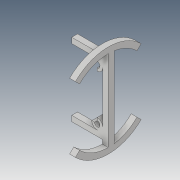
# Autodesk Inventor part: cameraMount2
Saved by Autodesk Inventor 2018 (Build 220112000, 112)
## iProperties
Created: 2020-02-12
Part Number: cameraMount2
Material: Generic
Document SubType Name: Modeling
Designer: anirudh.bali
Density: 1 g/cm^3
Appearance: Default
Author: anirudh.bali
Autodesk Inventor part; units mm, degrees
ref_plane "YZ Plane" through (0, 0, 0) normal (1, 0, 0) x (0, 1, 0)
ref_plane "XZ Plane" through (0, 0, 0) normal (0, 1, 0) x (-1, 0, 0)
ref_plane "XY Plane" through (0, 0, 0) normal (0, 0, 1) x (1, 0, 0)
sketch "Sketch2" plane through (0, 0, 0) normal (0, 0, 1) x (1, 0, 0)
  line L0 (0, 0) -> (40, 0)
  line L1 (40, 0) -> (40, 40)
  line L2 (40, 40) -> (0, 40)
  line L3 (0, 40) -> (0, 0)
  line L4 (0, 40) -> (2.5, 40)
  line L5 (40, 0) -> (37.5, 0)
  arc A0 (7.5046, 33.9954) -> (6.0046, 32.4954) centre (6.0046, 33.9954) ccw
  line L6 (6.0046, 32.4954) -> (6.0046, 30.9908)
  line L7 (7.5046, 33.9954) -> (9.0092, 33.9954)
  line L8 (0, 40) -> (3, 40)
  line L9 (40, 40) -> (37, 40)
  line L10 (0, 40) -> (3, 40)
  line L11 (40, 0) -> (37, 0)
  line L12 (6.0046, 37) -> (33.9954, 37)
  line L13 (37, 33.9954) -> (37, 6.0046)
  line L14 (33.9954, 3) -> (6.0046, 3)
  line L15 (3, 6.0046) -> (3, 33.9954)
  line L16 (20, 37) -> (6.0046, 37)
  line L17 (3, 20) -> (3, 33.9954)
  line L18 (7.5046, 33.9954) -> (9.0092, 33.9954)
  line L19 (6.0046, 30.9908) -> (6.0046, 32.4954)
  arc A1 (9.0092, 33.9954) -> (6.0046, 37) centre (6.0046, 33.9954) ccw
  arc A2 (3, 33.9954) -> (6.0046, 30.9908) centre (6.0046, 33.9954) ccw
  arc A3 (33.9954, 30.9908) -> (37, 33.9954) centre (33.9954, 33.9954) ccw
  line L20 (33.9954, 32.4954) -> (33.9954, 30.9908)
  arc A4 (33.9954, 32.4954) -> (32.4954, 33.9954) centre (33.9954, 33.9954) ccw
  line L21 (32.4954, 33.9954) -> (30.9908, 33.9954)
  arc A5 (33.9954, 37) -> (30.9908, 33.9954) centre (33.9954, 33.9954) ccw
  arc A6 (6.0046, 9.0092) -> (3, 6.0046) centre (6.0046, 6.0046) ccw
  line L22 (6.0046, 7.5046) -> (6.0046, 9.0092)
  arc A7 (6.0046, 7.5046) -> (7.5046, 6.0046) centre (6.0046, 6.0046) ccw
  line L23 (7.5046, 6.0046) -> (9.0092, 6.0046)
  arc A8 (6.0046, 3) -> (9.0092, 6.0046) centre (6.0046, 6.0046) ccw
  arc A9 (30.9908, 6.0046) -> (33.9954, 3) centre (33.9954, 6.0046) ccw
  arc A10 (32.4954, 6.0046) -> (33.9954, 7.5046) centre (33.9954, 6.0046) ccw
  line L24 (32.4954, 6.0046) -> (30.9908, 6.0046)
  line L25 (33.9954, 7.5046) -> (33.9954, 9.0092)
  arc A11 (37, 6.0046) -> (33.9954, 9.0092) centre (33.9954, 6.0046) ccw
  dimension "d3" = 3
  dimension "d4" = 3
  constraints: 52 end point, 24 point on circle, 12 centre point, 5 point on line, 4 horizontal, 4 parallel, 3 perpendicular, 2 midpoint, 1 vertical
  measures "d3" distance of L2.end L8.end
  measures "d4" distance of L0.end L11.end
extrude "Extrusion2" add sketch "Sketch2" along normal blind 3.175
sketch "Sketch4" plane through (40, 0, 0) normal (1, 0, 0) x (0, 0, -1)
  line L0 (-3.175, 6.0046) -> (-3.175, 33.9954) projected
  line L1 (0, 40) -> (-3.175, 40) projected
  line L2 (-3.175, 40) -> (-3.175, 45.4)
  line L3 (0, 0) -> (0, -5.2008)
  line L4 (-3.175, 0) -> (-3.175, 40) projected
  line L5 (0, 0) -> (0, 40) projected
  line L6 (-3.175, 40) -> (0, 40)
  line L7 (-3.175, 0) -> (0, 0)
  line L8 (-3.175, 45.4) -> (-3.175, 40)
  line L9 (-3.175, 0) -> (-3.175, -5.4)
  line L10 (0, -5.2008) -> (0, 0)
  line L11 (0, 40) -> (0, 45.2008)
  arc A0 (-3.175, -5.4) -> (0, -5.2008) centre (-3.175, 20) ccw
  arc A1 (0, 45.2008) -> (-3.175, 45.4) centre (-3.175, 20) ccw
  constraints: 16 end point, 4 point on circle, 2 centre point, 2 perpendicular, 1 horizontal, 1 midpoint, 1 vertical
extrude "Extrusion3" add sketch "Sketch4" against normal blind 40.005 contours L7 L3 A0 L9 | L2 A1 L11 L1
sketch "Sketch5" plane through (40, -5.4, 3.175) normal (1, 0, 0) x (0, 0, -1)
  line L0 (0, 39.3954) -> (0, 11.4046) projected
  arc A0 (3.175, 50.6008) -> (0, 50.8) centre (0, 25.4) ccw projected
  line L1 (0, 50.8) -> (0, 0) projected
  arc A1 (0, 0) -> (0, 50.8) centre (0, 25.4) ccw
  arc A2 (0, 3.175) -> (0, 47.625) centre (0, 25.4) ccw
  line L2 (0, 47.625) -> (0, 50.8)
  line L3 (0, 3.175) -> (0, 0)
  point P0 (3.175, 5.4)
  dimension "d13" = 44.45
  constraints: 4 end point, 4 point on circle, 2 centre point, 2 coincident, 2 point on line, 1 collinear, 1 vertical
  measures "d13" diameter of A2
extrude "Extrusion4" add sketch "Sketch5" against normal blind 3.175 contours L1 A0 A1 A2
ref_plane "Work Plane1" through (20, 0, 0) normal (-1, 0, 0) x (0, 0, 1)
mirror "Mirror1" about plane through (20, 0, 0) normal (-1, 0, 0) of "Extrusion4"
sketch "Sketch6" plane through (0, 0, 3.175) normal (0, 0, 1) x (1, 0, 0)
  line L0 (3.175, -1.997) -> (3.175, 41.997) projected
  line L1 (3.175, 41.997) -> (3.175, 45.4)
  line L2 (0, 41.997) -> (3.175, 41.997) projected
  line L3 (6.0046, 37) -> (33.9954, 37) projected
  line L4 (40, 45.4) -> (-0.005, 45.4) projected
  line L5 (36.825, 39.9972) -> (3.175, 39.9972)
  line L6 (3.175, 39.9972) -> (3.175, 45.4)
  line L7 (3.175, 45.4) -> (36.825, 45.4)
  line L8 (36.825, 45.4) -> (36.825, 39.9972)
  line L9 (36.825, -5.2008) -> (36.825, -5.4)
  line L10 (6.0046, 3) -> (33.9954, 3) projected
  line L11 (36.825, 0.0028) -> (3.175, 0.0028)
  line L12 (3.175, 0.0028) -> (3.175, -5.4)
  line L13 (3.175, -5.4) -> (36.825, -5.4)
  line L14 (36.825, -5.4) -> (36.825, 0.0028)
  point P0 (3, 6.0046)
  constraints: 20 end point, 4 parallel, 3 perpendicular, 2 horizontal, 1 point on line
extrude "Extrusion5" cut sketch "Sketch6" against normal blind 6.35
sketch "Sketch7" plane through (40, 20, 3.175) normal (1, 0, 0) x (0, 0, -1)
  line L0 (0, -13.9954) -> (0, 13.9954) projected
  arc A0 (3.6286, 25.1395) -> (0, 21.997) centre (3.175, 21.997) ccw projected
  line L1 (11.7893, 11.7893) -> (20.3814, 20.3814)
  line L2 (0, 0) -> (28.8237, 0) construction
  line L3 (11.7893, -11.7893) -> (20.3814, -20.3814)
  line L4 (0, 0) -> (33.8146, 0) construction
  arc A1 (20.3814, -20.3814) -> (20.3814, 20.3814) centre (0, 0) ccw
  line L5 (11.7893, 11.7893) -> (11.7893, -11.7893)
  point P0 (3.175, -20)
  dimension "d23" = 45
  dimension "d24" = 45
  constraints: 10 end point, 3 point on circle, 2 horizontal, 1 centre point, 1 coincident, 1 midpoint, 1 vertical
  measures "d23" angle of L2 L1
  measures "d24" angle of L3 L4
extrude "Extrusion6" cut sketch "Sketch7" against normal blind 61.9125
sketch "Sketch8" plane through (40, -5.4, 3.175) normal (1, 0, 0) x (0, 0, -1)
  line L0 (0, 11.4046) -> (0, 39.3954) projected
  arc A0 (17.9605, 43.3605) -> (0, 50.8) centre (0, 25.4) ccw projected
  line L1 (17.9605, 43.3605) -> (15.7154, 41.1154) projected
  line L2 (-15.7154, 41.1154) -> (-17.9605, 43.3605)
  line L3 (-15.7154, 9.6846) -> (-17.9605, 7.4395)
  line L4 (0, 47.625) -> (0, 50.8)
  line L5 (0, 50.8) -> (0, 47.625)
  line L6 (0, 3.175) -> (0, 0)
  arc A1 (-15.7154, 9.6846) -> (0, 3.175) centre (0, 25.4) ccw
  arc A2 (0, 47.625) -> (-15.7154, 41.1154) centre (0, 25.4) ccw
  arc A3 (-17.9605, 7.4395) -> (0, 0) centre (0, 25.4) ccw
  arc A4 (0, 50.8) -> (-17.9605, 43.3605) centre (0, 25.4) ccw
  point P0 (3.175, 5.4)
  constraints: 12 end point, 8 point on circle, 4 centre point, 1 coincident, 1 midpoint, 1 perpendicular, 1 vertical
extrude "Extrusion7" add sketch "Sketch8" against normal blind 3.175
sketch "Sketch9" plane through (0, 0, 0) normal (-1, 0, 0) x (0, 0, 1)
  line L0 (-20.0995, 50.6943) -> (25.4461, 50.6943)
  line L1 (25.4461, 50.6943) -> (25.4461, -10.2973)
  line L2 (25.4461, -10.2973) -> (-20.0995, -10.2973)
  line L3 (-20.0995, -10.2973) -> (-20.0995, 50.6943)
  point P0 (0, 0)
  constraints: 8 end point, 2 parallel, 1 horizontal, 1 perpendicular
extrude "Extrusion8" cut sketch "Sketch9" against normal blind 20.0025
sketch "Sketch10" plane through (-0.005, 0, 0) normal (-1, 0, 0) x (0, 0, 1)
  line L0 (-5.2888, 52.8999) -> (10.518, 52.8999)
  line L1 (10.518, 52.8999) -> (10.518, -9.6951)
  line L2 (10.518, -9.6951) -> (-5.2888, -9.6951)
  line L3 (-5.2888, -9.6951) -> (-5.2888, 52.8999)
  point P0 (0, 0)
  constraints: 8 end point, 2 parallel, 1 horizontal, 1 perpendicular
extrude "Extrusion9" cut sketch "Sketch10" along normal blind 12.7 and the other way blind 12.7
body "Solid2"
